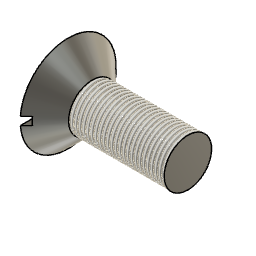
Screw_Jack_Assembly (Autodesk Fusion 360 archive; units mm, degrees)
design "screw"
Autodesk Fusion 360 part; units mm, degrees
sketch "Sketch1" plane through (0, 0, 0) normal (0, 1, 0) x (1, 0, 0)
sketch "Sketch2" plane through (0, 0, 0) normal (0, 1, 0) x (1, 0, 0)
  line L0 (0, 0) -> (0, -12)
  line L1 (0, -12) -> (6, -6)
  line L2 (6, -6) -> (6, 0)
  line L3 (0, 0) -> (30, 0)
  line L4 (6, -6) -> (30, -6)
  line L5 (30, -6) -> (30, 0)
  line L6 (30, 0) -> (6, 0)
  line L7 (6, 0) -> (6, -6)
  dimension "d1" = 12
  dimension "d4" = 30
  constraint coincident L0.start L3.start
  constraint vertical L0
  constraint perpendicular L0 L3
  constraint coincident L3 L2.end
  constraint horizontal L4
  constraint vertical L5
  constraint horizontal L6
  constraint vertical L7
  measures "d1" distance of L0.start L0.end
  measures "d4" distance of L0.start L3.end
revolve "Revolve1" add sketch "Sketch2" angle 360 about axis through (0, 0, 0) along (1, 0, 0)
sketch "Sketch3" plane through (0, 0, 0) normal (0, 1, 0) x (1, 0, 0)
  line L0 (1.5, 1) -> (-1.5, 1)
  line L1 (-1.5, 1) -> (-1.5, -1)
  line L2 (-1.5, -1) -> (1.5, -1)
  line L3 (1.5, -1) -> (1.5, 1)
  line L4 (1.5, 1) -> (-1.5, -1) construction
  line L5 (-1.5, 1) -> (1.5, -1) construction
  dimension "d6" = 3
  dimension "d7" = 2
  constraint horizontal L0
  constraint perpendicular L0 L1
  constraint parallel L0 L2
  constraint parallel L1 L3
  constraint coincident L4 origin
  constraint coincident L5 origin
  measures "d6" distance of L1.end L2.end
  measures "d7" distance of L0.end L1.end
extrude "Extrude1" cut sketch "Sketch3" along normal mid plane 400
thread "Thread1" "ISO Metric profile 12.0 M12x1 6g" major diameter 11.884 minor diameter 10.7405 pitch 1 angle 60 resizes the face on face at (14, 0.2991, 5.9925)

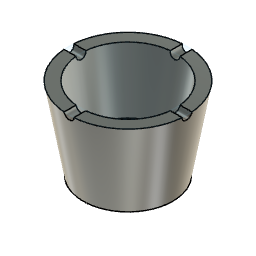
design "Untitled"
Autodesk Fusion 360 part; units mm, degrees
sketch "Sketch1" plane through (0, 0, 0) normal (0, 1, 0) x (1, 0, 0)
sketch "Sketch2" plane through (0, 0, 0) normal (0, 1, 0) x (1, 0, 0)
sketch "Sketch3" plane through (0, 0, 0) normal (0, 1, 0) x (1, 0, 0)
  line L0 (0, 0) -> (0, -42) construction
  line L1 (11, 0) -> (11, -12)
  line L2 (11, 0) -> (22.5, 0)
  line L3 (11, -12) -> (19, -12)
  line L4 (22.5, 0) -> (66.6999, 0) construction
  line L5 (30.1183, -40.5023) -> (24.9088, -10.9581)
  line L6 (19, -12) -> (24.2094, -41.5442)
  line L7 (24.9088, -10.9581) -> (22.9766, 0)
  line L8 (22.9766, 0) -> (22.5, 0)
  line L9 (24.2898, -42) -> (30.3824, -42)
  line L10 (24.2094, -41.5442) -> (24.2898, -42)
  line L11 (30.3824, -42) -> (30.1183, -40.5023)
  dimension "d1" = 42
  dimension "d2" = 11
  dimension "d4" = 22.5
  dimension "d8" = 6
  constraint coincident L0.start origin
  constraint vertical L0
  constraint vertical L1
  constraint perpendicular L1 L3
  constraint horizontal L4
  constraint coincident L4 L7.end
  constraint perpendicular L0 L9
  measures "d1" distance of L0.start L0.end
  measures "d2" distance of L0.start L1.start
  measures "d4" distance of L0.start L2.end
  measures "d8" distance of L6.end L5.start
revolve "Revolve1" add sketch "Sketch3" angle 360 about axis through (0, 0, 0) along (0, 0, 1)
sketch "Sketch4" plane through (0, 0, 42) normal (0, 0, 1) x (-1, 0, 0)
  circle A0 centre (0, 0) radius 30.3824
  circle A1 centre (0, 0) radius 24.2898
sketch "Sketch5" plane through (0, 0, 0) normal (0, 1, 0) x (1, 0, 0)
  line L0 (0, -42) -> (2.5, -42)
  arc A0 (2.5, -42) -> (0, -39.5) centre (0, -42) ccw
  arc A1 (0, -39.5) -> (-2.5, -42) centre (0, -42) ccw
  line L1 (-2.5, -42) -> (2.5, -42)
  dimension "d10" = 2.5
  dimension "d11" = 2.5
  constraint horizontal L0
  constraint parallel L0 L1
  measures "d10" distance of L0.start L0.end
  measures "d11" distance of L0.start A0.end
extrude "Extrude1" cut sketch "Sketch5" along normal mid plane 400
sketch "Sketch6" plane through (0, 0, 0) normal (1, 0, 0) x (0, 1, 0)
sketch "Sketch7" plane through (0, 0, 0) normal (1, 0, 0) x (0, 1, 0)
  line L0 (0, 42) -> (2.5, 42)
  arc A0 (0, 39.5) -> (2.5, 42) centre (0, 42) ccw
  arc A1 (-2.5, 42) -> (0, 39.5) centre (0, 42) ccw
  line L1 (-2.5, 42) -> (2.5, 42)
  line L2 (-2.5, 42) -> (2.5, 42)
  dimension "d15" = 2.5
  dimension "d16" = 2.5
  constraint horizontal L0
  constraint parallel L0 L1
  measures "d15" distance of L0.start L0.end
  measures "d16" distance of L0.start A0.start
extrude "Extrude2" cut sketch "Sketch7" along normal mid plane 400

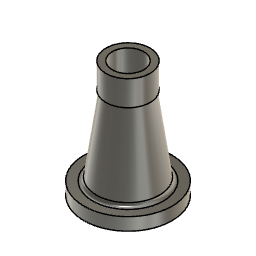
design "Body"
Autodesk Fusion 360 part; units mm, degrees
sketch "Sketch1" plane through (0, 0, 0) normal (0, 1, 0) x (1, 0, 0)
  line L0 (50, 0) -> (70, 0)
  line L1 (0, 0) -> (0, -3)
  line L2 (0, 0) -> (0, -185)
  line L3 (25, -185) -> (35, -185)
  line L4 (25, -185) -> (25, -145)
  line L5 (35, -185) -> (35, -145)
  line L6 (33, -145) -> (35, -145)
  line L7 (70, 0) -> (70, -20)
  line L8 (56, -20) -> (70, -20)
  arc A0 (56, -20) -> (50.0599, -25.1544) centre (56, -26) ccw
  line L9 (33, -145) -> (50.0599, -25.1544)
  line L10 (25, -175) -> (25, -155)
  line L11 (25, -130.2418) -> (40.1597, -23.7451)
  line L12 (43.1127, -3) -> (47, -3)
  line L13 (40.1597, -23.7451) -> (43.1127, -3)
  line L14 (25, -145) -> (25, -130.2418)
  arc A1 (47, -3) -> (50, 0) centre (47, 0) ccw
  dimension "d1" = 70
  dimension "d2" = 50
  dimension "d3" = 3
  dimension "d4" = 185
  dimension "d5" = 25
  dimension "d6" = 35
  dimension "d7" = 40
  dimension "d9" = 20
  dimension "d10" = 6
  dimension "d12" = 3
  constraint horizontal L0
  constraint coincident L1.start L2.start
  constraint perpendicular L0 L2
  constraint perpendicular L2 L3
  constraint perpendicular L3 L5
  constraint perpendicular L5 L6
  constraint perpendicular L0 L7
  constraint perpendicular L7 L8
  constraint tangent L8 A0
  constraint tangent A0 L9
  constraint perpendicular L2 L12
  constraint parallel L11 L13
  constraint parallel L4 L14
  constraint tangent L12 A1
  measures "d1" distance of L1.start L0.end
  measures "d2" distance of L1.start L0.start
  measures "d3" distance of L1.start L1.end
  measures "d4" distance of L1.start L2.end
  measures "d5" distance of L2.end L3.start
  measures "d6" distance of L2.end L3.end
  measures "d7" distance of L3.start L4.end
  measures "d9" distance of L0.end L7.end
  measures "d10" radius of A0
  measures "d12" radius of A1
revolve "Revolve1" add sketch "Sketch1" angle 360 about axis through (0, 0, 0) along (0, 0, 1)

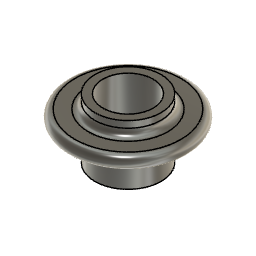
design "Untitled"
Autodesk Fusion 360 part; units mm, degrees
sketch "Sketch1" plane through (0, 0, 0) normal (0, 1, 0) x (1, 0, 0)
  line L0 (0, 0) -> (0, -45)
  line L1 (19, 0) -> (25, 0)
  line L2 (25, 0) -> (25, -25)
  line L3 (25, -25) -> (40, -25)
  line L4 (40, -35) -> (30, -35)
  line L5 (25, -40) -> (25, -45)
  line L6 (25, -45) -> (19, -45)
  line L7 (19, 0) -> (19, -45)
  arc A0 (30, -35) -> (25, -40) centre (30, -40) ccw
  arc A1 (40, -35) -> (40, -25) centre (40, -30) ccw
  dimension "d1" = 45
  dimension "d2" = 25
  dimension "d3" = 25
  dimension "d6" = 19
  dimension "d7" = 5
  dimension "d9" = 5
  constraint coincident L0.start origin
  constraint vertical L0
  constraint perpendicular L0 L1
  constraint perpendicular L1 L2
  constraint perpendicular L2 L3
  constraint perpendicular L2 L4
  constraint perpendicular L3 L5
  constraint perpendicular L0 L6
  constraint perpendicular L6 L7
  constraint tangent L5 A0
  constraint tangent L4 A0
  constraint tangent L4 A1
  constraint tangent L3 A1
  measures "d1" distance of L0.start L0.end
  measures "d2" distance of L0.start L1.end
  measures "d3" distance of L1.end L2.end
  measures "d6" distance of L0.start L1.start
  measures "d7" radius of A0
  measures "d9" radius of A1
revolve "Revolve1" add sketch "Sketch1" angle 360 about axis through (0, 0, 0) along (0, 0, 1)

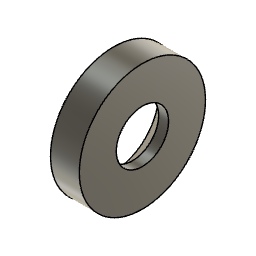
design "washer"
Autodesk Fusion 360 part; units mm, degrees
sketch "Sketch1" plane through (0, 0, 0) normal (0, 1, 0) x (1, 0, 0)
  line L0 (5.25, 0) -> (8, 0)
  line L1 (8, -7.25) -> (8, -17.5)
  line L2 (8, -7.25) -> (5.25, -7.25) construction
  line L3 (8, -17.5) -> (0, -17.5)
  line L4 (0, -12.5) -> (5.25, -7.25)
  line L5 (0, -17.5) -> (0, -12.5)
  line L6 (8, -7.25) -> (5.25, -7.25)
  dimension "d1" = 8
  dimension "d2" = 17.5
  dimension "d3" = 7.25
  dimension "d5" = 12.5
  constraint horizontal L0
  constraint perpendicular L0 L1
  constraint horizontal L2
  measures "d1" distance of origin L0.end
  measures "d2" distance of L0.end L1.end
  measures "d3" distance of L0.end L1.start
  measures "d5" distance of origin L4.start
revolve "Revolve1" add sketch "Sketch1" angle 360 about axis through (5.25, 0, 0) along (1, 0, 0)
equation "d2 = ( 35 / 2 ) * 1 mm"
equation "d3 = ( 14.5 / 2 ) * 1 mm"
equation "d5 = ( 25 / 2 ) * 1 mm"
